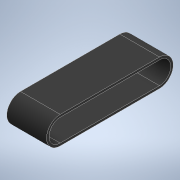
# Autodesk Inventor part: Conveyor Belt New
Saved by Autodesk Inventor 2022.2 (Build 262287000, 287)
## iProperties
Created: 2022-02-21
Part Number: Conveyor Belt New
Material: Rubber, Silicone
Document SubType Name: Modeling
Designer: PRASHANTH
Density: 1.25 g/cm^3
Appearance: Rubber - Black
Author: PRASHANTH
Autodesk Inventor part; units mm, degrees
ref_plane "YZ Plane" through (0, 0, 0) normal (1, 0, 0) x (0, 1, 0)
ref_plane "XZ Plane" through (0, 0, 0) normal (0, 1, 0) x (-1, 0, 0)
ref_plane "XY Plane" through (0, 0, 0) normal (0, 0, 1) x (1, 0, 0)
sketch "Sketch1" plane through (0, 0, 0) normal (1, 0, 0) x (0, 1, 0)
  line L0 (0, 100) -> (0, -100) construction
  line L1 (-22.5, 100) -> (-22.5, -100)
  line L2 (22.5, -100) -> (22.5, 100)
  arc A0 (22.5, 100) -> (-22.5, 100) centre (0, 100) ccw
  arc A1 (-22.5, -100) -> (22.5, -100) centre (0, -100) ccw
  line L3 (27.5, 100) -> (27.5, -100)
  arc A2 (-27.5, -100) -> (27.5, -100) centre (0, -100) ccw
  line L4 (-27.5, -100) -> (-27.5, 100)
  arc A3 (27.5, 100) -> (-27.5, 100) centre (0, 100) ccw
  point P0 (0, 0)
  dimension "d0" = 100
  dimension "d1" = 45
  dimension "d2" = 5
  constraints: 12 end point, 8 point on circle, 4 centre point, 4 tangent, 2 parallel, 1 midpoint, 1 vertical, 3 other
  measures "d0" distance of point (0, 0) L0.end
  measures "d1" diameter of A1
  measures "d2" distance between parallel lines of L2 L3
extrude "Extrusion1" add sketch "Sketch1" along normal blind 80
body "Solid1"
